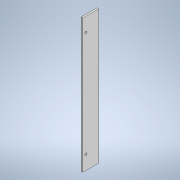
# Autodesk Inventor part: Template-Fixture-Side
Saved by Autodesk Inventor 2021 (Build 250183000, 183)
## iProperties
Created: 2020-06-15
Part Number: Template-Fixture-Side
Material: Generic
Document SubType Name: Modeling
Designer: lucas
Density: 1 g/cm^3
Appearance: Default
Project: 4Wire-FDM
Author: lucas
Revision Number: RLS_004
Autodesk Inventor part; units mm, degrees
ref_plane "YZ Plane" through (0, 0, 0) normal (1, 0, 0) x (0, 1, 0)
ref_plane "XZ Plane" through (0, 0, 0) normal (0, 1, 0) x (-1, 0, 0)
ref_plane "XY Plane" through (0, 0, 0) normal (0, 0, 1) x (1, 0, 0)
sketch "Sketch1" plane through (0, 0, 0) normal (1, 0, 0) x (0, 1, 0)
  circle A0 centre (99.0555, 7.2619) radius 1.6
  line L0 (99.0555, 7.2619) -> (-50.9445, 7.2619) construction
  line L1 (99.0555, 7.2619) -> (249.0555, 7.2619) construction
  circle A1 centre (-50.9445, 7.2619) radius 1.6
  circle A2 centre (99.0555, 7.2619) radius 1.6
  line L2 (99.0305, 11.4695) -> (119.0305, 11.4695)
  line L3 (119.0305, 11.4695) -> (119.0305, -11.2305)
  line L4 (119.0305, 11.4695) -> (141.7305, 11.4695) construction
  line L5 (119.0305, -11.2305) -> (-70.9695, -11.2305)
  line L6 (-70.9695, -11.2305) -> (-70.9695, 11.4695)
  line L7 (-70.9695, 11.4695) -> (99.0305, 11.4695)
  point P0 (0, 0)
  dimension "d0" = 150
  dimension "d1" = 180
  dimension "d2" = 3.2
  dimension "d3" = 3.2
  dimension "d4" = 20
  dimension "d5" = 22.7
  dimension "d6" = 90
  dimension "d7" = 190
  dimension "d8" = 90
  dimension "d9" = 22.7
  dimension "d10" = 90
  constraints: 16 end point, 4 horizontal, 3 centre point, 3 coincident, 2 equal length, 2 perpendicular, 1 vertical
  measures "d0" distance of L0.start L0.end
  measures "d1" angle of L0 L1
  measures "d2" diameter of A1
  measures "d3" diameter of A2
  measures "d4" distance of L2.start L2.end
  measures "d5" distance of L2.end L3.end
  measures "d6" angle of L3 L4
  measures "d7" distance of L3.end L5.end
  measures "d8" angle of L3 L5
  measures "d9" distance of L5.end L6.end
  measures "d10" angle of L5 L6
extrude "Extrusion1" add sketch "Sketch1" along normal blind 2.6
body "Solid1"
